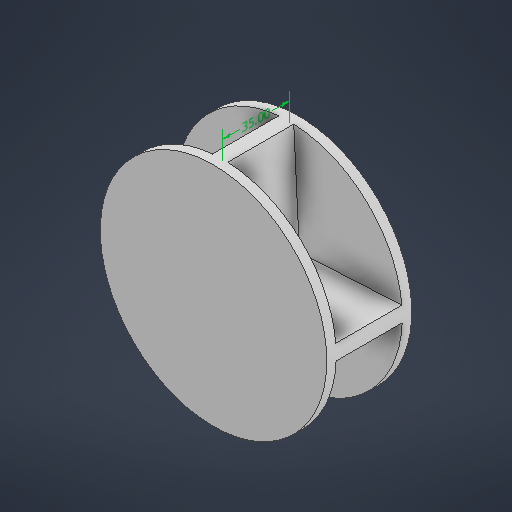
# Autodesk Inventor part: wheel
Saved by Autodesk Inventor 2026.2 (Build 302298000, 298)
## iProperties
Created: 2026-03-14
Part Number: wheel
Material: Generic
Document SubType Name: Modeling
Designer: danda
Density: 1 g/cm^3
Appearance: Default
Author: danda
Autodesk Inventor part; units mm, degrees
ref_plane "YZ Plane" through (0, 0, 0) normal (1, 0, 0) x (0, 1, 0)
ref_plane "XZ Plane" through (0, 0, 0) normal (0, 1, 0) x (-1, 0, 0)
ref_plane "XY Plane" through (0, 0, 0) normal (0, 0, 1) x (1, 0, 0)
sketch "Sketch1" plane through (0, 0, 0) normal (0, 0, 1) x (1, 0, 0)
  circle A0 centre (244.0918, 228.6255) radius 60
  line L0 (184.1439, 231.1255) -> (241.5918, 231.1255)
  line L1 (241.5918, 231.1255) -> (304.0397, 231.1255)
  line L2 (184.1439, 226.1255) -> (241.5918, 226.1255)
  line L3 (246.5918, 226.1255) -> (304.0397, 226.1255)
  line L4 (246.5918, 168.6776) -> (246.5918, 226.1255)
  line L5 (246.5918, 231.1255) -> (246.5918, 288.5734)
  line L6 (241.5918, 168.6776) -> (241.5918, 226.1255)
  line L7 (241.5918, 231.1255) -> (241.5918, 288.5734)
  arc A1 (294.0293, 231.1255) -> (246.5918, 278.5629) centre (244.0918, 228.6255) ccw
  arc A2 (246.5918, 178.688) -> (294.0293, 226.1255) centre (244.0918, 228.6255) ccw
  arc A3 (241.5918, 278.5629) -> (194.1544, 231.1255) centre (244.0918, 228.6255) ccw
  arc A4 (194.1544, 226.1255) -> (241.5918, 178.688) centre (244.0918, 228.6255) ccw
  line L8 (241.5918, 231.1255) -> (288.8318, 231.1255) construction
  line L9 (246.5918, 231.1255) -> (303.8392, 234.1257)
  line L10 (246.5918, 231.1255) -> (303.9178, 231.1255) construction
  line L11 (246.5918, 288.5734) -> (249.6026, 231.1255)
  line L12 (246.5918, 288.5734) -> (304.1186, 288.5734) construction
  line L13 (184.1439, 231.1255) -> (241.5918, 234.1362)
  line L14 (241.5918, 231.1255) -> (238.5916, 288.3728)
  line L15 (241.5918, 168.6776) -> (238.5811, 226.1255)
  line L16 (241.5918, 226.1255) -> (184.3445, 223.1253)
  line L17 (304.0397, 226.1255) -> (246.5918, 223.1147)
  line L18 (246.5918, 226.1255) -> (249.592, 168.8781)
  point P0 (0, 0)
  point P1 (246.7492, 223.123)
  point P2 (249.5943, 231.2828)
  point P3 (241.4345, 234.1279)
  point P4 (238.5894, 225.9681)
  dimension "d17" = 3
  dimension "d18" = 87
  dimension "d21" = 360
  constraints: 38 end point, 10 point on line, 8 parallel, 8 point on circle, 4 centre point, 3 horizontal, 2 equal length, 36 other
  measures "d17" angle of L10 L9
  measures "d18" angle of L11 L12
extrude "Extrusion1" add sketch "Sketch1" along normal blind 45
extrude "Extrusion2" cut sketch "Sketch1" along normal blind 40
extrude "Extrusion3" add sketch "Sketch1" along normal blind 40 contours A0 L3 L4 L6 L2 L0 L1 | L1 A1 L9 A0 | L17 A2 L3 | L1 L11 L9 A1 | A0 L4 A2 L18 | A2 L17 L18 L3 | L5 L1 L7 A0 | L11 A1 L5 | A2 L4 L17 L18 | L7 A3 L14 A0 | A1 L11 L9 L5 | L15 A4 L6 | L7 L13 L14 A3 | L0 A3 L13 L14 | A0 L2 A4 L16 | A4 L15 L16 L6 | L13 A3 L0 | A4 L2 L15 L16
extrude "Extrusion4" add sketch "Sketch1" along normal blind 5 contours A0 L18 A2 L17 | L9 A1 L11 A0 | A2 L18 L17 | L9 L11 A1 | A0 L16 A4 L15 | L14 A3 L13 A0 | A4 L16 L15 | L14 L13 A3
sketch "Sketch2" plane through (244.0918, 228.6255, 0) normal (0, 0, -1) x (-1, 0, 0)
  circle A0 centre (0, 0) radius 7.5
  point P0 (244.0918, -228.6255)
  dimension "d28" = 15
  constraints: 1 centre point
  measures "d28" diameter of A0
extrude "Extrusion5" cut sketch "Sketch2" against normal blind 10
body "Solid1"
